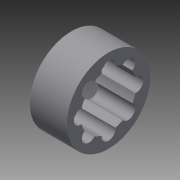
# Autodesk Inventor part: Ring1_NewDimensions_JacobMorgan_030215_pd3
Saved by Autodesk Inventor 2015 (Build 190159000, 159)
## iProperties
Created: 2015-03-02
Part Number: Ring1_NewDimensions_JacobMorgan_030215_pd3
Material: Generic
Document SubType Name: Modeling
Designer: WASHHSST
Density: 1 g/cm^3
Appearance: Default
Author: WASHHSST
Autodesk Inventor part; units mm, degrees
ref_plane "YZ Plane" through (0, 0, 0) normal (1, 0, 0) x (0, 1, 0)
ref_plane "XZ Plane" through (0, 0, 0) normal (0, 1, 0) x (-1, 0, 0)
ref_plane "XY Plane" through (0, 0, 0) normal (0, 0, 1) x (1, 0, 0)
sketch "Sketch7" plane through (0, 0, 0) normal (1, 0, 0) x (0, 1, 0)
  circle A0 centre (0, 0) radius 57.15
  circle A1 centre (0, 0) radius 38.1
  dimension "d24" = 114.3
  dimension "d25" = 76.2
  constraints: 2 centre point, 2 coincident
  measures "d24" diameter of A0
  measures "d25" diameter of A1
extrude "Extrusion6" add sketch "Sketch7" against normal blind 50.8
sketch "Sketch8" plane through (0, 0, 0) normal (1, 0, 0) x (0, 0, -1)
  circle A0 centre (0, 0) radius 38.1 projected
  circle A1 centre (0, 38.1) radius 9.525
  circle A2 centre (-26.9408, 26.9408) radius 9.525
  circle A3 centre (-38.1, 0) radius 9.525
  circle A4 centre (-26.9408, -26.9408) radius 9.525
  circle A5 centre (0, -38.1) radius 9.525
  circle A6 centre (26.9408, -26.9408) radius 9.525
  circle A7 centre (38.1, 0) radius 9.525
  circle A8 centre (26.9408, 26.9408) radius 9.525
  dimension "d28" = 19.05
  dimension "d31" = 360
  constraints: 8 centre point, 1 vertical alignment, 18 other
  measures "d28" diameter of A1
extrude "Extrusion7" cut sketch "Sketch8" against normal blind 76.2 contours A0 A7 | A0 A7 | A8 A0 | A0 A8 | A6 A0 | A0 A6 | A1 A0 | A0 A1 | A5 A0 | A0 A5 | A2 A0 | A0 A2 | A4 A0 | A0 A4 | A3 A0 | A0 A3
body "Solid2"
